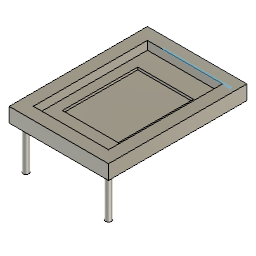
PolarFrame (Autodesk Fusion 360 design; units mm, degrees)
part number: 2025-10-05-21-01-06-559
Autodesk Fusion 360 part; units mm, degrees
sketch "Sketch1" plane through (0, 0, 0) normal (0, 0, 1) x (1, 0, 0)
  line L0 (0, 0) -> (54, 0)
  line L1 (54, 0) -> (54, 86)
  line L2 (54, 86) -> (0, 86)
  line L3 (0, 86) -> (0, 0)
  line L4 (0, 0) -> (4, 0)
  line L5 (54, 0) -> (50, 0)
  line L6 (2.5994, 86) -> (2.5994, 78) construction
  line L7 (0, 81.5035) -> (4, 81.5035) construction
  line L8 (4.0277, 78.0304) -> (50.0277, 78.0304)
  line L9 (50.0277, 78.0304) -> (50.0277, 16.0304)
  line L10 (50.0277, 16.0304) -> (4.0277, 16.0304)
  line L11 (4.0277, 16.0304) -> (4.0277, 78.0304)
  line L12 (58.8409, 16.0304) -> (58.8409, 0) construction
  line L13 (50.0277, 78.0304) -> (50.0277, 94.0304) construction
  line L14 (50.0277, 78.0304) -> (58.0277, 78.0304) construction
  line L15 (58.0277, 94.0304) -> (-3.9723, 94.0304)
  line L16 (-3.9723, 94.0304) -> (-3.9723, 0.0304)
  line L17 (-3.9723, 0.0304) -> (58.0277, 0.0304)
  line L18 (58.0277, 0.0304) -> (58.0277, 94.0304)
  line L19 (-3.9723, 94.0304) -> (-13.9723, 94.0304) construction
  line L20 (-13.9723, 94.0304) -> (-13.9723, 104.0304) construction
  line L21 (-13.9723, 104.0304) -> (68.0277, 104.0304)
  line L22 (68.0277, 104.0304) -> (68.0277, -9.9696)
  line L23 (68.0277, -9.9696) -> (-13.9723, -9.9696)
  line L24 (-13.9723, -9.9696) -> (-13.9723, 104.0304)
  line L25 (0, 0) -> (-0.5, 0) construction
  line L26 (54, 0) -> (54.5, 0) construction
  line L27 (54.5, 0) -> (-0.5, 0)
  line L28 (-0.5, 0) -> (-0.5, 86)
  line L29 (-0.5, 86) -> (54.5, 86)
  line L30 (54.5, 86) -> (54.5, 0)
  line L31 (58.0277, 0.0304) -> (68.0277, 0.0304) construction
  dimension "d1" = 54
  dimension "d2" = 86
  dimension "d5" = 8
  dimension "d6" = 4
  dimension "d9" = 62
  dimension "d10" = 16
  dimension "d11" = 8
  dimension "d12" = 62
  dimension "d13" = 94
  dimension "d14" = 10
  dimension "d15" = 10
  dimension "d16" = 82
  dimension "d17" = 114
  dimension "d26" = 0.5
  dimension "d27" = 0.5
  dimension "d28" = 55
  constraint horizontal L0
  constraint vertical L1
  constraint horizontal L2
  constraint vertical L3
  constraint coincident L0.start L3.end
  constraint perpendicular L3 L4
  constraint perpendicular L1 L5
  constraint coincident L2 L6.start
  constraint perpendicular L2 L6
  constraint coincident L3 L7.start
  constraint perpendicular L3 L7
  constraint horizontal L8
  constraint vertical L9
  constraint horizontal L10
  constraint vertical L11
  constraint coincident L10 L12.start
  constraint coincident L0 L12.end
  constraint perpendicular L0 L12
  constraint perpendicular L8 L13
  constraint perpendicular L9 L14
  constraint horizontal L15
  constraint vertical L16
  constraint horizontal L17
  constraint vertical L18
  constraint perpendicular L16 L19
  constraint perpendicular L19 L20
  constraint horizontal L21
  constraint vertical L22
  constraint horizontal L23
  constraint vertical L24
  constraint perpendicular L3 L25
  constraint perpendicular L1 L26
  constraint horizontal L27
  constraint vertical L28
  constraint horizontal L29
  constraint vertical L30
  constraint coincident L22 L31.end
  constraint perpendicular L22 L31
  measures "d1" distance of L0.start L0.end
  measures "d2" distance of L0.start L2.end
  measures "d5" distance of L6.start L6.end
  measures "d6" distance of L7.start L7.end
  measures "d9" distance of L8.start L10.end
  measures "d10" distance of L8.end L13.end
  measures "d11" distance of L8.end L14.end
  measures "d12" distance of L15.start L15.end
  measures "d13" distance of L15.start L17.end
  measures "d14" distance of L15.end L19.end
  measures "d15" distance of L19.end L20.end
  measures "d16" distance of L20.end L21.end
  measures "d17" distance of L20.end L23.end
  measures "d26" distance of L0.start L25.end
  measures "d27" distance of L0.end L26.end
  measures "d28" distance of L26.end L25.end
extrude "Extrude1" add sketch "Sketch1" along normal blind 10 contours L0 L1 L3 L4 L5 L17 L27 | L3 L17 L27 L28 | L1 L17 L27 L30 | L21 L22 L23 L24
extrude "Extrude2" cut sketch "Sketch1" along normal blind 1 contours L0 L1 L3 L4 L5 L17 L27 | L3 L17 L27 L28 | L3 L17 L28 L29 | L1 L2 L3 L17 L29 | L2 L15 L16 L17 L18 L28 L29 L30 | L1 L17 L27 L30 | L1 L17 L29 L30 | L8 L9 L10 L11 | L21 L22 L23 L24
extrude "Extrude3" add sketch "Sketch1" along normal blind 1 and the other way blind 1 contours L0 L1 L3 L4 L5 L17 L27 | L3 L17 L27 L28 | L3 L17 L28 L29 | L1 L2 L3 L17 L29 | L2 L15 L16 L17 L18 L28 L29 L30 | L1 L17 L27 L30 | L1 L17 L29 L30 | L8 L9 L10 L11 | L21 L22 L23 L24
extrude "Extrude4" add 1 faces at (13.361, 66.0304, -1) along direction (0, 0, -1) blind 1
extrude "Extrude5" add sketch "Sketch1" against normal blind 2 contours L3 L17 L28 L29 | L1 L2 L3 L17 L29 | L2 L15 L16 L17 L18 L28 L29 L30 | L1 L17 L29 L30 | L8 L9 L10 L11
sketch "Sketch2" plane through (0, 104.0304, 0) normal (0, 1, 0) x (-1, 0, 0)
  line L0 (13.9723, -2) -> (13.9723, 10)
  line L1 (13.9723, 10) -> (-68.0277, 10)
  line L2 (-68.0277, 10) -> (-68.0277, -2)
  line L3 (-68.0277, -2) -> (13.9723, -2)
  line L4 (0.5, 0) -> (-54.5, 0)
  line L5 (-54.5, 0) -> (-54.5, 1)
  line L6 (0.5, 0) -> (0.5, 1)
  line L7 (0.5, 1) -> (-54.5, 1)
  dimension "d35" = 55
  dimension "d55" = 1
  dimension "d56" = 1
  constraint horizontal L4
  constraint perpendicular L4 L5
  constraint perpendicular L4 L6
  measures "d35" distance of L4.start L4.end
  measures "d55" distance of L4.end L5.end
  measures "d56" distance of L4.start L6.end
extrude "Extrude6" add sketch "Sketch1" along normal blind 3 contours L2 L15 L16 L17 L18 L28 L29 L30
extrude "Extrude7" add sketch "Sketch1" along normal blind 2.5 from surface at 0.5 contours L3 L17 L28 L29 | L1 L2 L3 L17 L29 | L1 L17 L29 L30
extrude "Extrude8" cut sketch "Sketch2" against normal blind 29 contours L4 L5 L6 L7
sketch "Sketch3" plane through (0, 0, -2) normal (0, 0, -1) x (1, 0, 0)
  line L0 (68.0277, 9.9696) -> (-13.9723, 9.9696)
  line L1 (-13.9723, 9.9696) -> (-13.9723, -104.0304)
  line L2 (-13.9723, -104.0304) -> (68.0277, -104.0304)
  line L3 (68.0277, -104.0304) -> (68.0277, 9.9696)
  line L4 (68.0277, 9.9696) -> (61.0277, 9.9696) construction
  line L5 (-13.9723, 9.9696) -> (-6.9723, 9.9696) construction
  line L6 (61.0277, 9.9696) -> (61.0277, 2.9696) construction
  line L7 (-6.9723, 9.9696) -> (-6.9723, 2.9696) construction
  circle A0 centre (61.0277, 2.9696) radius 2.5
  circle A1 centre (-6.9723, 2.9696) radius 2.5
  dimension "d45" = 7
  dimension "d46" = 7
  dimension "d47" = 7
  dimension "d48" = 7
  dimension "d49" = 5
  dimension "d50" = 5
  constraint coincident L0.start L3.end
  constraint perpendicular L3 L4
  constraint coincident L0.end L1.start
  constraint perpendicular L1 L5
  constraint perpendicular L4 L6
  constraint perpendicular L5 L7
  constraint coincident L6.end A0.centre
  constraint coincident L7.end A1.centre
  measures "d45" distance of L0.start L4.end
  measures "d46" distance of L0.end L5.end
  measures "d47" distance of L4.end L6.end
  measures "d48" distance of L5.end L7.end
  measures "d49" diameter of A0
  measures "d50" diameter of A1
extrude "Extrude9" add sketch "Sketch3" along normal blind 35 contours A0
extrude "Extrude10" add sketch "Sketch3" along normal blind 35 contours A1
extrude "Extrude11" cut sketch "Sketch2" against normal blind 104 contours L4 L5 L6 L7
